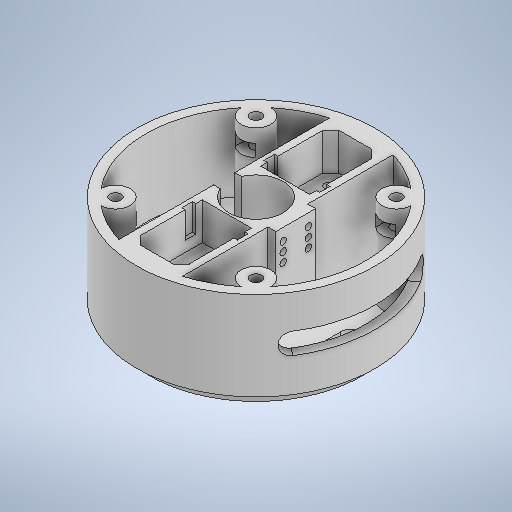
# Autodesk Inventor part: SCARA swivel top
Saved by Autodesk Inventor 2025.2 (Build 292293000, 293)
## iProperties
Created: 2025-01-26
Part Number: SCARA swivel top
Material: Generic
Document SubType Name: Modeling
Designer: caomi
Density: 1 g/cm^3
Appearance: Default
Author: caomi
Autodesk Inventor part; units mm, degrees
ref_plane "YZ Plane" through (0, 0, 0) normal (1, 0, 0) x (0, 1, 0)
ref_plane "XZ Plane" through (0, 0, 0) normal (0, 1, 0) x (-1, 0, 0)
ref_plane "XY Plane" through (0, 0, 0) normal (0, 0, 1) x (1, 0, 0)
sketch "Sketch1" plane through (0, 0, 0) normal (0, 1, 0) x (-1, 0, 0)
  circle A0 centre (0, 0) radius 45
  line L0 (9.25, 37.5) -> (-9.25, 37.5)
  line L1 (-9.25, 37.5) -> (-9.25, 11)
  line L2 (-9.25, 11) -> (9.25, 11)
  line L3 (9.25, 11) -> (9.25, 37.5)
  line L4 (-9.25, -11) -> (9.25, -11)
  line L5 (9.25, -11) -> (9.25, -37.5)
  line L6 (9.25, -37.5) -> (-9.25, -37.5)
  line L7 (-9.25, -37.5) -> (-9.25, -11)
  line L8 (22.2209, 0) -> (-22.2209, 0) construction
  circle A1 centre (0, 0) radius 3
  circle A2 centre (0, 0) radius 10.25
  line L9 (-15.5, -15.5) -> (15.5, -15.5) construction
  line L10 (15.5, -15.5) -> (15.5, 15.5) construction
  line L11 (15.5, 15.5) -> (-15.5, 15.5) construction
  line L12 (-15.5, 15.5) -> (-15.5, -15.5) construction
  line L13 (-15.5, -15.5) -> (15.5, 15.5) construction
  line L14 (15.5, -15.5) -> (-15.5, 15.5) construction
  line L15 (0, 48.862) -> (0, 10.8876) construction
  line L16 (0, -56.5383) -> (0, 11.5383) construction
  circle A3 centre (15.5, 15.5) radius 1.5
  circle A4 centre (15.5, -15.5) radius 1.5
  circle A5 centre (-15.5, -15.5) radius 1.5
  circle A6 centre (-15.5, 15.5) radius 1.5
  line L17 (-4, -27.8627) -> (-0.85, -29.6813)
  line L18 (-0.85, -29.6813) -> (-0.85, -33.3187)
  line L19 (-0.85, -33.3187) -> (-4, -35.1373)
  line L20 (-4, -35.1373) -> (-7.15, -33.3187)
  line L21 (-7.15, -33.3187) -> (-7.15, -29.6813)
  line L22 (-7.15, -29.6813) -> (-4, -27.8627)
  line L23 (4, -27.8627) -> (7.15, -29.6813)
  line L24 (7.15, -29.6813) -> (7.15, -33.3187)
  line L25 (7.15, -33.3187) -> (4, -35.1373)
  line L26 (4, -35.1373) -> (0.85, -33.3187)
  line L27 (0.85, -33.3187) -> (0.85, -29.6813)
  line L28 (0.85, -29.6813) -> (4, -27.8627)
  line L29 (-4, 27.8627) -> (-0.85, 29.6813)
  line L30 (-0.85, 29.6813) -> (-0.85, 33.3187)
  line L31 (-0.85, 33.3187) -> (-4, 35.1373)
  line L32 (-4, 35.1373) -> (-7.15, 33.3187)
  line L33 (-7.15, 33.3187) -> (-7.15, 29.6813)
  line L34 (-7.15, 29.6813) -> (-4, 27.8627)
  line L35 (4, 27.8627) -> (7.15, 29.6813)
  line L36 (7.15, 29.6813) -> (7.15, 33.3187)
  line L37 (7.15, 33.3187) -> (4, 35.1373)
  line L38 (4, 35.1373) -> (0.85, 33.3187)
  line L39 (0.85, 33.3187) -> (0.85, 29.6813)
  line L40 (0.85, 29.6813) -> (4, 27.8627)
  circle A7 centre (-4, -31.5) radius 1.65
  circle A8 centre (4, -31.5) radius 1.65
  circle A9 centre (-4, 31.5) radius 1.65
  circle A10 centre (4, 31.5) radius 1.65
  point P0 (0, 22.5)
  point P1 (0, -22.5)
  point P2 (0, -22.5)
  point P3 (-0.85, -31.5)
  dimension "d0" = 90
  dimension "d11" = 6
  dimension "d12" = 20.5
  dimension "d13" = 31
  dimension "d15" = 18.5
  dimension "d16" = 15
  dimension "d17" = 15
  dimension "d18" = 45
  dimension "d19" = 3
  dimension "d23" = 8
  dimension "d25" = 3.3
  dimension "d70" = 9
  dimension "d71" = 26.5
  dimension "d72" = 6.3
  constraints: 82 end point, 18 symmetric about line, 11 centre point, 9 coincident, 6 parallel, 5 midpoint, 4 equal length, 4 equal radius, 4 horizontal, 4 vertical, 3 perpendicular, 2 point on line, 2 vertical alignment, 1 horizontal alignment, 30 other
  measures "d0" diameter of A0
  measures "d11" diameter of A1
  measures "d12" diameter of A2
  measures "d13" distance of L9.end L10.end
  measures "d15" distance of L0.start L0.end
  measures "d16" distance from line of L0 point (0, 22.5)
  measures "d17" distance from line of point (0, -22.5) L6
  measures "d18" distance of point (0, -22.5) point (0, 22.5)
  measures "d19" diameter of A3
  measures "d23" distance of point (-4, -31.5) point (4, -31.5)
  measures "d25" diameter of A7
  measures "d70" vertical distance of point (0, -22.5) point (-4, -31.5)
  measures "d71" distance of L6.end L4.start
  measures "d72" distance from line of point (-0.85, -31.5) L21
extrude "Base" add sketch "Sketch1" against normal blind 15 contours A0 | L3 L2 L1 L0 | L4 L5 L6 L7 | A2 | A3 | A4 | A5 | A6
extrude "M3 nut stop" add sketch "Sketch1" against normal blind 3 contours L17 L18 L19 L20 L21 L22 | L23 L24 L25 L26 L27 L28 | L34 L33 L32 L31 L30 L29 | L40 L39 L38 L37 L36 L35
extrude "Top" add sketch "Sketch1" along normal blind 20.5 contours A0
extrude "Base of shaft support" add sketch "Sketch1" along normal blind 6.5 contours L3 L2 L1 L0 | L4 L5 L6 L7 | L17 L18 L19 L20 L21 L22 | L23 L24 L25 L26 L27 L28 | L34 L33 L32 L31 L30 L29 | L40 L39 L38 L37 L36 L35
chamfer "Corners of shaft support" distance 3 angle 45 4 edges at (-9.25, 13.5, 37.5) (9.25, 13.5, 37.5) (-9.25, 13.5, -37.5) (9.25, 13.5, -37.5)
extrude "Stepper mount holes" cut sketch "Sketch1" along normal through all both and the other way through all contours A3 | A4 | A5 | A6
sketch "Sketch4" plane through (0, -15, 0) normal (0, -1, 0) x (1, 0, 0)
  circle A0 centre (0, 0) radius 11
  dimension "d34" = 22
  constraints: 1 centre point, 1 coincident
  measures "d34" diameter of A0
extrude "Stepper face mount" cut sketch "Sketch4" against normal blind 2
sketch "Sketch5" plane through (0, 20.5, 0) normal (0, 1, 0) x (1, 0, 0)
  circle A0 centre (0, 0) radius 3 projected
  circle A1 centre (0, 0) radius 41.5
  line L0 (-12, -39.7272) -> (-12, 39.7272)
  line L1 (12, 39.7272) -> (12, -39.7272)
  line L2 (0, 51.8199) -> (0, 0) construction
  circle A2 centre (0, 0) radius 45 projected
  dimension "d38" = 12
  dimension "d76" = 3.5
  constraints: 6 end point, 4 point on circle, 3 vertical, 1 centre point, 1 coincident, 1 other
  measures "d38" distance between parallel lines of L1 L2
  measures "d76" radial gap between concentric circles of A2 A1
extrude "Material reduction" cut sketch "Sketch5" against normal blind 34 contours A1 L1 | L0 A1
sketch "Sketch6" plane through (0, 20.5, 0) normal (0, 1, 0) x (1, 0, 0)
  circle A0 centre (-26.5165, 26.5165) radius 5.5
  line L0 (-26.5165, 26.5165) -> (0, 0) construction
  line L1 (-23.7305, 0) -> (26.8317, 0) construction
  circle A1 centre (-26.5165, -26.5165) radius 5.5
  line L2 (-26.5165, -26.5165) -> (0, 0) construction
  line L3 (0, 17.9751) -> (0, -18.8342) construction
  circle A2 centre (26.5165, 26.5165) radius 5.5
  circle A3 centre (26.5165, -26.5165) radius 5.5
  line L4 (-22.7665, 24.3514) -> (-26.5165, 22.1864)
  line L5 (-26.5165, 22.1864) -> (-30.2665, 24.3514)
  line L6 (-30.2665, 24.3514) -> (-30.2665, 28.6816)
  line L7 (-30.2665, 28.6816) -> (-26.5165, 30.8466)
  line L8 (-26.5165, 30.8466) -> (-22.7665, 28.6816)
  line L9 (-22.7665, 28.6816) -> (-22.7665, 24.3514)
  circle A4 centre (-26.5165, 26.5165) radius 2.05
  line L10 (0, -17.9751) -> (0, 18.8342) construction
  line L11 (-22.7665, -24.3514) -> (-26.5165, -22.1864)
  line L12 (-26.5165, -22.1864) -> (-30.2665, -24.3514)
  line L13 (-30.2665, -24.3514) -> (-30.2665, -28.6816)
  line L14 (-30.2665, -28.6816) -> (-26.5165, -30.8466)
  line L15 (-26.5165, -30.8466) -> (-22.7665, -28.6816)
  line L16 (-22.7665, -28.6816) -> (-22.7665, -24.3514)
  circle A5 centre (-26.5165, -26.5165) radius 2.05
  line L17 (22.7665, 24.3514) -> (26.5165, 22.1864)
  line L18 (26.5165, 22.1864) -> (30.2665, 24.3514)
  line L19 (30.2665, 24.3514) -> (30.2665, 28.6816)
  line L20 (30.2665, 28.6816) -> (26.5165, 30.8466)
  line L21 (26.5165, 30.8466) -> (22.7665, 28.6816)
  line L22 (22.7665, 28.6816) -> (22.7665, 24.3514)
  circle A6 centre (26.5165, 26.5165) radius 2.05
  line L23 (30.2665, -28.6816) -> (26.5165, -30.8466)
  line L24 (30.2665, -24.3514) -> (30.2665, -28.6816)
  line L25 (26.5165, -22.1864) -> (30.2665, -24.3514)
  circle A7 centre (26.5165, -26.5165) radius 2.05
  line L26 (22.7665, -24.3514) -> (26.5165, -22.1864)
  line L27 (22.7665, -28.6816) -> (22.7665, -24.3514)
  line L28 (26.5165, -30.8466) -> (22.7665, -28.6816)
  line L29 (-30.2665, 24.3514) -> (-30.2665, 22.4931)
  line L30 (-22.7665, 24.3514) -> (-22.7665, 22.4931)
  line L31 (-30.2665, -24.3514) -> (-30.2665, -22.4931)
  line L32 (-22.7665, -24.3514) -> (-22.7665, -22.4931)
  line L33 (30.2665, 24.3514) -> (30.2665, 22.4931)
  line L34 (22.7665, 24.3514) -> (22.7665, 22.4931)
  line L35 (30.2665, -24.3514) -> (30.2665, -22.4931)
  line L36 (22.7665, -24.3514) -> (22.7665, -22.4931)
  point P0 (22.7665, 22.4931)
  point P1 (30.2665, 22.4931)
  point P2 (30.2665, -22.4931)
  point P3 (22.7665, -22.4931)
  point P4 (-22.7665, -22.4931)
  point P5 (-30.2665, -22.4931)
  dimension "d41" = 37.5
  dimension "d43" = 11
  dimension "d44" = 45
  dimension "d45" = 7.5
  dimension "d46" = 4.1
  constraints: 74 end point, 31 symmetric about line, 8 centre point, 2 coincident, 2 collinear, 2 point on circle, 2 vertical, 1 equal radius, 1 horizontal, 1 point on line, 20 other
  measures "d41" distance of L0.start L0.end
  measures "d43" diameter of A0
  measures "d44" angle of L1 L0
  measures "d45" distance between parallel lines of L8 L5
  measures "d46" diameter of A4
extrude "Slot for M4 fasteners" add sketch "Sketch6" against normal up to surface (34 mm away)
ref_plane "Work Plane1" through (0, 15.5, 0) normal (0, 1, 0) x (1, 0, 0)
extrude "Slot for M4 nuts to fasen to the swivel base" cut sketch "Sketch6" against normal blind 4.7 from surface at -5 contours L29 L5 L4 L30 A0 | L6 L7 L8 L9 L4 L5 | L32 L11 L12 L31 A1 | L16 L15 L14 L13 L12 L11 | L34 L17 L18 L33 A2 | L22 L21 L20 L19 L18 L17 | L35 L25 L26 L36 A3 | L24 L23 L28 L27 L26 L25
sketch "Sketch7" plane through (0, -13.5, 0) normal (0, 1, 0) x (1, 0, 0)
  line L0 (-18.5591, 0) -> (20.3221, 0) construction
  line L1 (12, -39.7272) -> (12, 39.7272) projected
  line L2 (12, 7.5) -> (15, 7.5)
  line L3 (15, 7.5) -> (15, -7.5)
  line L4 (15, -7.5) -> (12, -7.5)
  line L5 (12, -7.5) -> (12, 7.5)
  point P0 (0, 0)
  dimension "d61" = 15
  dimension "d62" = 3
  constraints: 10 end point, 2 horizontal, 2 parallel, 2 point on line, 1 perpendicular, 1 other
  measures "d61" distance of L2.end L3.end
  measures "d62" distance between parallel lines of L1 L3
extrude "Mounting face for limit switch" add sketch "Sketch7" along normal up to surface (34 mm away)
sketch "Sketch8" plane through (15, -13.5, -7.5) normal (-1, 0, 0) x (0, 0, 1)
  circle A0 centre (12.25, 26) radius 1.2
  circle A1 centre (2.75, 26) radius 1.2
  line L0 (2.75, 26) -> (12.25, 26) construction
  line L1 (7.5, 28.9581) -> (7.5, 20.5932) construction
  line L2 (0, 34) -> (15, 34) projected
  circle A2 centre (12.25, 29.5) radius 1.2
  circle A3 centre (2.75, 29.5) radius 1.2
  circle A4 centre (12.25, 22.5) radius 1.2
  circle A5 centre (2.75, 22.5) radius 1.2
  point P0 (7.5, 13.5)
  point P1 (7.5, 34)
  dimension "d56" = 9.5
  dimension "d57" = 2.4
  dimension "d63" = 8
  dimension "d86" = 3.5
  dimension "d89" = 3.5
  constraints: 6 centre point, 4 end point, 3 equal radius, 2 vertical, 2 vertical alignment, 1 horizontal, 1 horizontal alignment, 1 midpoint, 1 point on line, 5 other
  measures "d56" distance of L0.start L0.end
  measures "d57" diameter of A1
  measures "d63" distance between parallel lines of L0 L2
  measures "d86" distance of L0.end A2.centre
  measures "d89" distance of L0.end A4.centre
extrude "Mounting holes for limit switch" cut sketch "Sketch8" along normal blind 3.5
sketch "Sketch9" plane through (0, -15, 0) normal (0, -1, 0) x (1, 0, 0)
  line L0 (-21.25, -21.25) -> (21.25, -21.25)
  line L1 (21.25, -21.25) -> (21.25, 21.25)
  line L2 (21.25, 21.25) -> (-21.25, 21.25)
  line L3 (-21.25, 21.25) -> (-21.25, -21.25)
  line L4 (-21.25, -21.25) -> (21.25, 21.25) construction
  line L5 (21.25, -21.25) -> (-21.25, 21.25) construction
  circle A0 centre (0, 0) radius 45 projected
  line L6 (7.15, 33.3187) -> (7.15, 29.6813) projected
  line L7 (0.85, 29.6813) -> (0.85, 33.3187) projected
  line L8 (4, 27.8627) -> (0.85, 29.6813) projected
  line L9 (7.15, 29.6813) -> (4, 27.8627) projected
  line L10 (0.85, 33.3187) -> (4, 35.1373) projected
  line L11 (4, 35.1373) -> (7.15, 33.3187) projected
  line L12 (-0.85, 33.3187) -> (-0.85, 29.6813) projected
  line L13 (-4, 35.1373) -> (-0.85, 33.3187) projected
  line L14 (-7.15, 33.3187) -> (-4, 35.1373) projected
  line L15 (-7.15, 29.6813) -> (-7.15, 33.3187) projected
  line L16 (-4, 27.8627) -> (-7.15, 29.6813) projected
  line L17 (-0.85, 29.6813) -> (-4, 27.8627) projected
  circle A1 centre (-15.5, 15.5) radius 1.5 projected
  circle A2 centre (15.5, 15.5) radius 1.5 projected
  circle A3 centre (15.5, -15.5) radius 1.5 projected
  circle A4 centre (0, 0) radius 11 projected
  circle A5 centre (15.5, 15.5) radius 1.5 projected
  circle A6 centre (-15.5, 15.5) radius 1.5 projected
  circle A7 centre (15.5, -15.5) radius 1.5 projected
  circle A8 centre (-15.5, -15.5) radius 1.5 projected
  circle A9 centre (0, 0) radius 45 projected
  line L18 (7.15, 33.3187) -> (7.15, 29.6813) projected
  line L19 (7.15, 29.6813) -> (4, 27.8627) projected
  line L20 (4, 27.8627) -> (0.85, 29.6813) projected
  line L21 (0.85, 29.6813) -> (0.85, 33.3187) projected
  line L22 (0.85, 33.3187) -> (4, 35.1373) projected
  line L23 (4, 35.1373) -> (7.15, 33.3187) projected
  line L24 (-7.15, 29.6813) -> (-7.15, 33.3187) projected
  line L25 (-7.15, 33.3187) -> (-4, 35.1373) projected
  line L26 (-4, 35.1373) -> (-0.85, 33.3187) projected
  line L27 (-0.85, 33.3187) -> (-0.85, 29.6813) projected
  line L28 (-0.85, 29.6813) -> (-4, 27.8627) projected
  line L29 (-4, 27.8627) -> (-7.15, 29.6813) projected
  line L30 (0.85, -29.6813) -> (4, -27.8627) projected
  line L31 (4, -27.8627) -> (7.15, -29.6813) projected
  line L32 (7.15, -29.6813) -> (7.15, -33.3187) projected
  line L33 (7.15, -33.3187) -> (4, -35.1373) projected
  line L34 (4, -35.1373) -> (0.85, -33.3187) projected
  line L35 (0.85, -33.3187) -> (0.85, -29.6813) projected
  line L36 (-7.15, -29.6813) -> (-4, -27.8627) projected
  line L37 (-4, -27.8627) -> (-0.85, -29.6813) projected
  line L38 (-0.85, -29.6813) -> (-0.85, -33.3187) projected
  line L39 (-0.85, -33.3187) -> (-4, -35.1373) projected
  line L40 (-4, -35.1373) -> (-7.15, -33.3187) projected
  line L41 (-7.15, -33.3187) -> (-7.15, -29.6813) projected
  dimension "d64" = 42.5
  constraints: 12 end point, 2 midpoint, 2 parallel, 2 perpendicular, 1 horizontal
  measures "d64" distance of L1.end L2.end
extrude "Recess face for stepper mounting" add sketch "Sketch9" along normal blind 3 contours A0
chamfer "Corner of stepper mounting face" distance 3.5 angle 45 4 edges at (21.25, -16.5, 21.25) (21.25, -16.5, -21.25) (-21.25, -16.5, -21.25) (-21.25, -16.5, 21.25)
chamfer "Material reduction at the base" distance 5 angle 45 7 edges at (-45, -18, 0) (41.5, -13.5, 0) (19.5862, -13.5, 36.5873) (19.5862, -13.5, -36.5873) (-19.5862, -13.5, 36.5873) (-41.5, -13.5, 0) (-19.5862, -13.5, -36.5873)
sketch "Sketch10" plane through (0, -13.5, 0) normal (0, 1, 0) x (1, 0, 0)
  line L0 (30, 6) -> (30, -6) construction
  line L1 (26, 6) -> (26, -6)
  line L2 (34, -6) -> (34, 6)
  arc A0 (34, 6) -> (26, 6) centre (30, 6) ccw
  arc A1 (26, -6) -> (34, -6) centre (30, -6) ccw
  point P0 (0, 0)
  point P1 (30, 0)
  dimension "d77" = 12
  dimension "d78" = 30
  dimension "d79" = 4
  constraints: 8 end point, 4 point on circle, 4 tangent, 2 centre point, 1 horizontal alignment, 1 midpoint, 1 parallel, 1 vertical
  measures "d77" distance of L0.start L0.end
  measures "d78" distance from line of point (0, 0) L0
  measures "d79" radius of A1
extrude "Wiring slot 1" cut sketch "Sketch10" against normal up to next
sketch "Sketch11" plane through (0, 0, 0) normal (0, 0, 1) x (1, 0, 0)
  line L0 (49, 7.75) -> (41, 7.75)
  line L1 (41, 7.75) -> (41, -0.25)
  line L2 (41, -0.25) -> (49, -0.25)
  line L3 (49, -0.25) -> (49, 7.75)
  line L4 (45, 20.5) -> (45, -13) construction
  line L5 (45, 20.5) -> (45, -13) construction
  line L6 (0, -19.7) -> (0, 27.2) projected
  point P0 (0, 0)
  point P1 (49, 3.75)
  point P2 (45, 3.75)
  point P3 (45, 7.75)
  dimension "d82" = 8
  dimension "d83" = 8
  constraints: 10 end point, 3 midpoint, 3 point on line, 2 parallel, 1 horizontal, 1 horizontal alignment, 1 perpendicular
  measures "d82" distance of L0.start L0.end
  measures "d83" distance of L2.end L0.start
revolve "Wiring slot 2" cut sketch "Sketch11" angle 75 mid plane about axis through (0, -10, 0) along (0, 1, 0)
fillet "Fillet1" radius 4 4 edges at (34.3125, 7.75, 26.3289) (34.3125, -0.25, 26.3289) (34.3125, 7.75, -26.3289) (34.3125, -0.25, -26.3289)
sketch "Sketch12" plane through (-12, 20.5, -39.7272) normal (-1, 0, 0) x (0, 0, 1)
  line L0 (43.7272, -20.5) -> (35.7272, -20.5)
  line L1 (35.7272, -20.5) -> (35.7272, 0)
  line L2 (35.7272, 0) -> (43.7272, 0)
  line L3 (43.7272, 0) -> (43.7272, -20.5)
  line L4 (43.7272, -20.5) -> (35.7272, 0) construction
  line L5 (35.7272, -20.5) -> (43.7272, 0) construction
  line L6 (0, 0) -> (79.4544, 0) projected
  line L7 (49.9772, -20.5) -> (29.4772, -20.5) projected
  point P0 (39.7272, -20.5)
  point P1 (39.7272, -10.25)
  point P2 (39.7272, 0)
  dimension "d94" = 8
  constraints: 12 end point, 3 midpoint, 2 collinear, 2 parallel, 1 horizontal, 1 perpendicular, 1 vertical alignment
  measures "d94" distance of L0.start L0.end
extrude "Screwing slot" cut sketch "Sketch12" against normal up to surface round surface about axis through (0, 0, 0) along (0, 1, 0) radius 10.25 far side no
chamfer "Chamfer4" distance 2 angle 45 2 edges at (-10.7186, 0, 4) (-10.7186, 0, -4)
sketch "Sketch13" plane through (0, 20.5, 0) normal (0, 1, 0) x (1, 0, 0)
  line L0 (10.5, -17.5) -> (-10.5, -17.5)
  line L1 (-10.5, -17.5) -> (-10.5, -13.5)
  line L2 (-10.5, -13.5) -> (10.5, -13.5)
  line L3 (10.5, -13.5) -> (10.5, -17.5)
  line L4 (10.5, -17.5) -> (-10.5, -13.5) construction
  line L5 (-10.5, -17.5) -> (10.5, -13.5) construction
  line L6 (-9.25, -11) -> (9.25, -11) projected
  circle A0 centre (4, -31.5) radius 1.65 projected
  point P0 (0, 0)
  point P1 (0, -15.5)
  point P2 (0, -11)
  dimension "d100" = 4
  dimension "d101" = 21
  dimension "d102" = 16
  constraints: 12 end point, 3 midpoint, 2 parallel, 1 horizontal, 1 perpendicular, 1 vertical alignment
  measures "d100" distance of L0.end L1.end
  measures "d101" distance of L1.end L2.end
  measures "d102" vertical distance of A0.centre point (0, -15.5)
extrude "Extrusion15" cut sketch "Sketch13" against normal blind 10 contours L0 L1 L2 L3
mirror "Mirror1" about plane through (0, 0, 0) normal (0, 0, 1) of "Extrusion15"
body "Solid1"
